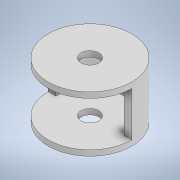
# Autodesk Inventor part: Rubberfoot
Saved by Autodesk Inventor 2022 (Build 260153000, 153)
## iProperties
Created: 2021-12-09
Part Number: Rubberfoot
Material: Genérico
Document SubType Name: Modeling
Designer: JK
Density: 1 g/cm^3
Appearance: Valor por defecto
Author: JK
Autodesk Inventor part; units mm, degrees
ref_plane "YZ Plane" through (0, 0, 0) normal (1, 0, 0) x (0, 1, 0)
ref_plane "XZ Plane" through (0, 0, 0) normal (0, 1, 0) x (-1, 0, 0)
ref_plane "XY Plane" through (0, 0, 0) normal (0, 0, 1) x (1, 0, 0)
sketch "Boceto1" plane through (0, 0, 0) normal (0, 1, 0) x (-1, 0, 0)
  circle A0 centre (0, 0) radius 7.5
  dimension "d0" = 15
  constraints: 1 centre point, 1 coincident
  measures "d0" diameter of A0
extrude "Extrusión1" add sketch "Boceto1" along normal mid plane 10
sketch "Boceto2" plane through (0, 0, 0) normal (0, 1, 0) x (-1, 0, 0)
  circle A0 centre (0, 0) radius 6.15
  dimension "d3" = 12.3
  constraints: 1 centre point, 1 coincident
  measures "d3" diameter of A0
extrude "Extrusión2" cut sketch "Boceto2" along normal mid plane 8
sketch "Boceto3" plane through (0, 5, 0) normal (0, 1, 0) x (1, 0, 0)
  circle A0 centre (0, 0) radius 1.6
  dimension "d6" = 3.2
  constraints: 1 centre point, 1 coincident
  measures "d6" diameter of A0
extrude "Extrusión3" cut sketch "Boceto3" against normal through all
sketch "Boceto4" plane through (0, 0, 0) normal (0, 0, 1) x (1, 0, 0)
  line L0 (-10.1106, -4) -> (10.1106, -4)
  line L1 (10.1106, -4) -> (10.1106, 4)
  line L2 (10.1106, 4) -> (-10.1106, 4)
  line L3 (-10.1106, 4) -> (-10.1106, -4)
  line L4 (-10.1106, -4) -> (10.1106, 4) construction
  line L5 (10.1106, -4) -> (-10.1106, 4) construction
  line L6 (-7.5, -5) -> (7.5, -5) projected
  point P0 (0, 0)
  dimension "d11" = 8
  dimension "d12" = 1
  constraints: 12 end point, 2 midpoint, 2 parallel, 1 horizontal, 1 perpendicular
  measures "d11" distance of L0.end L1.end
  measures "d12" distance between parallel lines of L0 L6
extrude "Extrusión4" cut sketch "Boceto4" along normal through all
